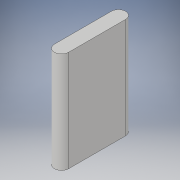
# Autodesk Inventor part: Cuerpo - Batería
Saved by Autodesk Inventor 2019 (Build 230136000, 136)
## iProperties
Created: 2020-03-12
Part Number: Cuerpo - Batería
Material: Generic
Document SubType Name: Modeling
Designer: Sanoli
Density: 1 g/cm^3
Appearance: Default
Author: Sanoli
Autodesk Inventor part; units mm, degrees
ref_plane "YZ Plane" through (0, 0, 0) normal (1, 0, 0) x (0, 1, 0)
ref_plane "XZ Plane" through (0, 0, 0) normal (0, 1, 0) x (-1, 0, 0)
ref_plane "XY Plane" through (0, 0, 0) normal (0, 0, 1) x (1, 0, 0)
sketch "Sketch1" plane through (0, 0, 0) normal (0, 1, 0) x (-1, 0, 0)
  arc A0 (14, 0) -> (0, 0) centre (7, 0) ccw
  line L0 (0, 0) -> (0, -56.5)
  line L1 (14, 0) -> (14, -56.5)
  arc A1 (0, -56.5) -> (14, -56.5) centre (7, -56.5) ccw
  dimension "d1" = 14
  dimension "d2" = 70.5
  constraints: 4 end point, 4 point on circle, 4 tangent, 2 centre point, 2 vertical
  measures "d1" distance between parallel lines of L1 L0
extrude "Extrusion1" add sketch "Sketch1" along normal blind 100
body "Solid1"
